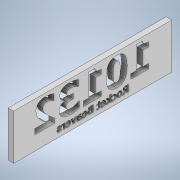
# Autodesk Inventor part: Vehicle Registration Plate
Saved by Autodesk Inventor 2020 (Build 240168000, 168)
## iProperties
Created: 2020-01-13
Part Number: Vehicle Registration Plate
Material: Generic
Document SubType Name: Modeling
Designer: maple
Density: 1 g/cm^3
Appearance: Default
Author: maple
Autodesk Inventor part; units mm, degrees
ref_plane "YZ Plane" through (0, 0, 0) normal (1, 0, 0) x (0, 1, 0)
ref_plane "XZ Plane" through (0, 0, 0) normal (0, 1, 0) x (-1, 0, 0)
ref_plane "XY Plane" through (0, 0, 0) normal (0, 0, 1) x (1, 0, 0)
sketch "Sketch1" plane through (0, 0, 0) normal (1, 0, 0) x (0, 1, 0)
  line L0 (0, 0) -> (-50.8, 0)
  line L1 (-50.8, 0) -> (-50.8, -177.8)
  line L2 (-50.8, -177.8) -> (0, -177.8)
  line L3 (0, -177.8) -> (0, 0)
  dimension "d0" = 50.8
  dimension "d1" = 177.8
  constraints: 8 end point, 2 parallel, 1 horizontal, 1 perpendicular
  measures "d0" distance of L2.end L1.end
  measures "d1" distance of L1.end L0.end
extrude "Extrusion1" add sketch "Sketch1" along normal blind 6.35
sketch "Sketch3" plane through (0, 0, 0) normal (-1, 0, 0) x (0, 0, 1)
  line L0 (-177.8, 0) -> (0, 0) projected
  line L1 (-88.9, 0) -> (-88.9, -50.8)
  line L2 (0, -50.8) -> (-177.8, -50.8) projected
  line L3 (-177.8, -50.8) -> (-177.8, 0) projected
  line L4 (-177.8, -25.4) -> (0, -25.4)
  line L5 (0, 0) -> (0, -50.8) projected
  line L6 (-172.4509, 0.5134) -> (-5.5704, 0.5134) construction
  line L7 (-5.5704, 0.5134) -> (-5.5704, -39.1921) construction
  line L8 (-5.5704, -39.1921) -> (-172.4509, -39.1921) construction
  line L9 (-172.4509, -39.1921) -> (-172.4509, 0.5134) construction
  line L10 (-156.8284, -35.0682) -> (-21.0393, -35.0682) construction
  line L11 (-21.0393, -35.0682) -> (-21.0393, -48.6327) construction
  line L12 (-21.0393, -48.6327) -> (-156.8284, -48.6327) construction
  line L13 (-156.8284, -48.6327) -> (-156.8284, -35.0682) construction
  line L14 (-131.6308, -34.5794) -> (-151.7614, -34.5794)
  line L15 (-151.7614, -34.5794) -> (-151.7614, -29.2688)
  line L16 (-151.7614, -29.2688) -> (-145.3394, -29.2688)
  line L17 (-145.3394, -29.2688) -> (-145.3394, -13.1396)
  line L18 (-145.3394, -13.1396) -> (-151.7614, -13.1396)
  line L19 (-151.7614, -13.1396) -> (-151.7614, -8.1749)
  spline S0 degree 2 poles (-151.7614, -8.1749) (-150.3535, -8.1749) (-147.5624, -7.8044) (-146.7226, -7.4092) knots 0 0 0 1 2 2 2
  spline S1 degree 2 poles (-146.7226, -7.4092) (-145.7593, -6.9152) (-144.6725, -5.2603) (-144.5737, -4.0253) knots 0 0 0 1 2 2 2
  line L20 (-144.5737, -4.0253) -> (-137.9046, -4.0253)
  line L21 (-137.9046, -4.0253) -> (-137.9046, -29.2688)
  line L22 (-137.9046, -29.2688) -> (-131.6308, -29.2688)
  line L23 (-131.6308, -29.2688) -> (-131.6308, -34.5794)
  spline S2 degree 2 poles (-103.9666, -19.3394) (-103.9666, -23.2914) (-105.2263, -29.2194) (-106.6342, -31.2201) knots 0 0 0 1 2 2 2
  spline S3 degree 2 poles (-106.6342, -31.2201) (-108.0174, -33.1962) (-112.4882, -35.2216) (-115.6992, -35.2216) knots 0 0 0 1 2 2 2
  spline S4 degree 2 poles (-115.6992, -35.2216) (-118.9349, -35.2216) (-123.3809, -33.1962) (-124.7889, -31.1707) knots 0 0 0 1 2 2 2
  spline S5 degree 2 poles (-124.7889, -31.1707) (-126.1968, -29.17) (-127.4565, -23.2914) (-127.4565, -19.3394) knots 0 0 0 1 2 2 2
  spline S6 degree 2 poles (-127.4565, -19.3394) (-127.4565, -15.2885) (-126.1968, -9.5581) (-124.7642, -7.4833) knots 0 0 0 1 2 2 2
  spline S7 degree 2 poles (-124.7642, -7.4833) (-123.3315, -5.4579) (-118.8114, -3.4819) (-115.6992, -3.4819) knots 0 0 0 1 2 2 2
  spline S8 degree 2 poles (-115.6992, -3.4819) (-112.4141, -3.4819) (-108.0174, -5.5567) (-106.6095, -7.6068) knots 0 0 0 1 2 2 2
  spline S9 degree 2 poles (-106.6095, -7.6068) (-105.2263, -9.6075) (-103.9666, -15.5108) (-103.9666, -19.3394) knots 0 0 0 1 2 2 2
  spline S10 degree 2 poles (-111.6484, -19.3394) (-111.6484, -13.683) (-113.5009, -9.1135) (-115.6992, -9.1135) knots 0 0 0 1 2 2 2
  spline S11 degree 2 poles (-115.6992, -9.1135) (-117.8975, -9.1135) (-119.7747, -13.683) (-119.7747, -19.3641) knots 0 0 0 1 2 2 2
  spline S12 degree 2 poles (-119.7747, -19.3641) (-119.7747, -24.9463) (-117.8975, -29.5899) (-115.6992, -29.5899) knots 0 0 0 1 2 2 2
  spline S13 degree 2 poles (-115.6992, -29.5899) (-113.5256, -29.5899) (-111.6484, -24.9463) (-111.6484, -19.3394) knots 0 0 0 1 2 2 2
  line L24 (-78.229, -34.5794) -> (-98.3597, -34.5794)
  line L25 (-98.3597, -34.5794) -> (-98.3597, -29.2688)
  line L26 (-98.3597, -29.2688) -> (-91.9376, -29.2688)
  line L27 (-91.9376, -29.2688) -> (-91.9376, -13.1396)
  line L28 (-91.9376, -13.1396) -> (-98.3597, -13.1396)
  line L29 (-98.3597, -13.1396) -> (-98.3597, -8.1749)
  spline S14 degree 2 poles (-98.3597, -8.1749) (-96.9518, -8.1749) (-94.1606, -7.8044) (-93.3208, -7.4092) knots 0 0 0 1 2 2 2
  spline S15 degree 2 poles (-93.3208, -7.4092) (-92.3575, -6.9152) (-91.2707, -5.2603) (-91.1719, -4.0253) knots 0 0 0 1 2 2 2
  line L30 (-91.1719, -4.0253) -> (-84.5029, -4.0253)
  line L31 (-84.5029, -4.0253) -> (-84.5029, -29.2688)
  line L32 (-84.5029, -29.2688) -> (-78.229, -29.2688)
  line L33 (-78.229, -29.2688) -> (-78.229, -34.5794)
  spline S16 degree 2 poles (-50.9354, -25.3415) (-50.9354, -27.5892) (-52.5903, -31.2695) (-54.1958, -32.5539) knots 0 0 0 1 2 2 2
  spline S17 degree 2 poles (-54.1958, -32.5539) (-55.8013, -33.8384) (-60.1732, -35.2216) (-63.3101, -35.2216) knots 0 0 0 1 2 2 2
  spline S18 degree 2 poles (-63.3101, -35.2216) (-66.867, -35.2216) (-71.9552, -34.036) (-73.5607, -33.295) knots 0 0 0 1 2 2 2
  line L34 (-73.5607, -33.295) -> (-73.5607, -26.6753)
  line L35 (-73.5607, -26.6753) -> (-72.8197, -26.6753)
  spline S19 degree 2 poles (-72.8197, -26.6753) (-71.1401, -27.7374) (-66.62, -29.3182) (-64.7428, -29.3182) knots 0 0 0 1 2 2 2
  spline S20 degree 2 poles (-64.7428, -29.3182) (-63.6312, -29.3182) (-61.0377, -28.923) (-60.1485, -28.2808) knots 0 0 0 1 2 2 2
  spline S21 degree 2 poles (-60.1485, -28.2808) (-59.4569, -27.7621) (-58.6171, -26.2554) (-58.6171, -24.8969) knots 0 0 0 1 2 2 2
  spline S22 degree 2 poles (-58.6171, -24.8969) (-58.6171, -23.5384) (-59.8027, -22.0811) (-60.7907, -21.7353) knots 0 0 0 1 2 2 2
  spline S23 degree 2 poles (-60.7907, -21.7353) (-61.7787, -21.3895) (-64.5205, -21.3154) (-65.5826, -21.3154) knots 0 0 0 1 2 2 2
  line L36 (-65.5826, -21.3154) -> (-66.8917, -21.3154)
  line L37 (-66.8917, -21.3154) -> (-66.8917, -15.9554)
  line L38 (-66.8917, -15.9554) -> (-65.6814, -15.9554)
  spline S24 degree 2 poles (-65.6814, -15.9554) (-64.2982, -15.9554) (-61.9516, -15.7084) (-61.1365, -15.3379) knots 0 0 0 1 2 2 2
  spline S25 degree 2 poles (-61.1365, -15.3379) (-60.3214, -14.9427) (-59.4075, -13.5595) (-59.4075, -12.3739) knots 0 0 0 1 2 2 2
  spline S26 degree 2 poles (-59.4075, -12.3739) (-59.4075, -11.4353) (-60.272, -10.2744) (-60.8895, -9.9533) knots 0 0 0 1 2 2 2
  spline S27 degree 2 poles (-60.8895, -9.9533) (-61.6305, -9.5828) (-63.6065, -9.3358) (-64.2982, -9.3358) knots 0 0 0 1 2 2 2
  spline S28 degree 2 poles (-64.2982, -9.3358) (-65.4097, -9.3358) (-67.7562, -9.8545) (-68.843, -10.2744) knots 0 0 0 1 2 2 2
  spline S29 degree 2 poles (-68.843, -10.2744) (-69.7075, -10.5955) (-71.5847, -11.6329) (-72.0293, -11.9046) knots 0 0 0 1 2 2 2
  line L39 (-72.0293, -11.9046) -> (-72.6715, -11.9046)
  line L40 (-72.6715, -11.9046) -> (-72.6715, -5.3838)
  spline S30 degree 2 poles (-72.6715, -5.3838) (-71.0907, -4.7169) (-65.7555, -3.4572) (-62.9643, -3.4572) knots 0 0 0 1 2 2 2
  spline S31 degree 2 poles (-62.9643, -3.4572) (-60.2473, -3.4572) (-56.2459, -4.3958) (-54.838, -5.3097) knots 0 0 0 1 2 2 2
  spline S32 degree 2 poles (-54.838, -5.3097) (-53.2819, -6.273) (-51.7258, -9.237) (-51.7258, -11.0895) knots 0 0 0 1 2 2 2
  spline S33 degree 2 poles (-51.7258, -11.0895) (-51.7258, -13.7077) (-54.7392, -17.6104) (-57.2092, -18.1785) knots 0 0 0 1 2 2 2
  line L41 (-57.2092, -18.1785) -> (-57.2092, -18.4749)
  spline S34 degree 2 poles (-57.2092, -18.4749) (-56.1224, -18.6231) (-54.0476, -19.4135) (-53.0596, -20.3027) knots 0 0 0 1 2 2 2
  spline S35 degree 2 poles (-53.0596, -20.3027) (-52.1457, -21.0931) (-50.9354, -23.6125) (-50.9354, -25.3415) knots 0 0 0 1 2 2 2
  line L42 (-23.4688, -34.5794) -> (-45.8718, -34.5794)
  line L43 (-45.8718, -34.5794) -> (-45.8718, -29.6146)
  spline S36 degree 2 poles (-45.8718, -29.6146) (-43.0313, -27.3422) (-38.4865, -23.3408) (-36.7822, -21.5377) knots 0 0 0 1 2 2 2
  spline S37 degree 2 poles (-36.7822, -21.5377) (-34.5345, -19.1912) (-32.5337, -15.6096) (-32.5337, -13.7324) knots 0 0 0 1 2 2 2
  spline S38 degree 2 poles (-32.5337, -13.7324) (-32.5337, -11.6082) (-35.0779, -9.3358) (-37.3503, -9.3358) knots 0 0 0 1 2 2 2
  spline S39 degree 2 poles (-37.3503, -9.3358) (-38.5112, -9.3358) (-40.586, -9.9039) (-41.6481, -10.3485) knots 0 0 0 1 2 2 2
  spline S40 degree 2 poles (-41.6481, -10.3485) (-42.6855, -10.8178) (-44.1675, -11.8058) (-44.538, -12.0528) knots 0 0 0 1 2 2 2
  line L44 (-44.538, -12.0528) -> (-45.1308, -12.0528)
  line L45 (-45.1308, -12.0528) -> (-45.1308, -5.4085)
  spline S41 degree 2 poles (-45.1308, -5.4085) (-43.8464, -4.791) (-38.363, -3.5066) (-35.8189, -3.5066) knots 0 0 0 1 2 2 2
  spline S42 degree 2 poles (-35.8189, -3.5066) (-30.3848, -3.5066) (-24.8026, -8.3478) (-24.8026, -12.7197) knots 0 0 0 1 2 2 2
  spline S43 degree 2 poles (-24.8026, -12.7197) (-24.8026, -15.412) (-27.3467, -20.5991) (-30.286, -23.5631) knots 0 0 0 1 2 2 2
  spline S44 degree 2 poles (-30.286, -23.5631) (-32.1385, -25.3909) (-35.6213, -28.2314) (-36.387, -28.8242) knots 0 0 0 1 2 2 2
  line L46 (-36.387, -28.8242) -> (-23.4688, -28.8242)
  line L47 (-23.4688, -28.8242) -> (-23.4688, -34.5794)
  line L48 (-121.8406, -45.7407) -> (-124.1686, -45.7407)
  line L49 (-124.1686, -45.7407) -> (-126.2866, -42.9434)
  line L50 (-126.2866, -42.9434) -> (-126.9783, -42.9434)
  line L51 (-126.9783, -42.9434) -> (-126.9783, -45.7407)
  line L52 (-126.9783, -45.7407) -> (-128.8802, -45.7407)
  line L53 (-128.8802, -45.7407) -> (-128.8802, -38.1207)
  line L54 (-128.8802, -38.1207) -> (-125.8173, -38.1207)
  spline S45 degree 2 poles (-125.8173, -38.1207) (-125.1813, -38.1207) (-124.2427, -38.2813) (-123.8413, -38.5283) knots 0 0 0 1 2 2 2
  spline S46 degree 2 poles (-123.8413, -38.5283) (-123.4338, -38.7876) (-122.9521, -39.5965) (-122.9521, -40.214) knots 0 0 0 1 2 2 2
  spline S47 degree 2 poles (-122.9521, -40.214) (-122.9521, -41.0847) (-123.7425, -42.1777) (-124.4033, -42.4988) knots 0 0 0 1 2 2 2
  line L55 (-124.4033, -42.4988) -> (-121.8406, -45.7407)
  spline S48 degree 2 poles (-124.9158, -40.4549) (-124.9158, -40.1646) (-125.1381, -39.7509) (-125.3913, -39.6398) knots 0 0 0 1 2 2 2
  spline S49 degree 2 poles (-125.3913, -39.6398) (-125.5703, -39.5657) (-126.0088, -39.5224) (-126.336, -39.5224) knots 0 0 0 1 2 2 2
  line L56 (-126.336, -39.5224) -> (-126.9783, -39.5224)
  line L57 (-126.9783, -39.5224) -> (-126.9783, -41.5726)
  line L58 (-126.9783, -41.5726) -> (-126.4287, -41.5726)
  spline S50 degree 2 poles (-126.4287, -41.5726) (-126.0335, -41.5726) (-125.4715, -41.4737) (-125.2801, -41.3194) knots 0 0 0 1 2 2 2
  spline S51 degree 2 poles (-125.2801, -41.3194) (-125.0949, -41.1712) (-124.9158, -40.776) (-124.9158, -40.4549) knots 0 0 0 1 2 2 2
  spline S52 degree 2 poles (-115.8632, -42.8693) (-115.8632, -44.2896) (-117.4131, -45.9198) (-118.8272, -45.9198) knots 0 0 0 1 2 2 2
  spline S53 degree 2 poles (-118.8272, -45.9198) (-120.2351, -45.9198) (-121.7974, -44.2896) (-121.7974, -42.8693) knots 0 0 0 1 2 2 2
  spline S54 degree 2 poles (-121.7974, -42.8693) (-121.7974, -41.4367) (-120.2351, -39.8127) (-118.8272, -39.8127) knots 0 0 0 1 2 2 2
  spline S55 degree 2 poles (-118.8272, -39.8127) (-117.4193, -39.8127) (-115.8632, -41.4429) (-115.8632, -42.8693) knots 0 0 0 1 2 2 2
  spline S56 degree 2 poles (-117.6972, -42.8817) (-117.6972, -42.3691) (-117.8639, -41.6837) (-118.0121, -41.4799) knots 0 0 0 1 2 2 2
  spline S57 degree 2 poles (-118.0121, -41.4799) (-118.1726, -41.2638) (-118.574, -41.0971) (-118.8272, -41.0971) knots 0 0 0 1 2 2 2
  spline S58 degree 2 poles (-118.8272, -41.0971) (-119.0742, -41.0971) (-119.4632, -41.2453) (-119.6238, -41.4552) knots 0 0 0 1 2 2 2
  spline S59 degree 2 poles (-119.6238, -41.4552) (-119.7782, -41.6528) (-119.9634, -42.3506) (-119.9634, -42.8817) knots 0 0 0 1 2 2 2
  spline S60 degree 2 poles (-119.9634, -42.8817) (-119.9634, -43.4065) (-119.7905, -44.0549) (-119.6485, -44.2525) knots 0 0 0 1 2 2 2
  spline S61 degree 2 poles (-119.6485, -44.2525) (-119.5065, -44.4501) (-119.0742, -44.6354) (-118.8148, -44.6354) knots 0 0 0 1 2 2 2
  spline S62 degree 2 poles (-118.8148, -44.6354) (-118.5987, -44.6354) (-118.1541, -44.4501) (-118.0183, -44.2649) knots 0 0 0 1 2 2 2
  spline S63 degree 2 poles (-118.0183, -44.2649) (-117.8639, -44.0487) (-117.6972, -43.4251) (-117.6972, -42.8817) knots 0 0 0 1 2 2 2
  spline S64 degree 2 poles (-112.0964, -45.8951) (-112.8065, -45.8951) (-113.986, -45.5369) (-114.4244, -45.1664) knots 0 0 0 1 2 2 2
  spline S65 degree 2 poles (-114.4244, -45.1664) (-114.8505, -44.7897) (-115.3321, -43.6597) (-115.3321, -42.894) knots 0 0 0 1 2 2 2
  spline S66 degree 2 poles (-115.3321, -42.894) (-115.3321, -42.0666) (-114.8134, -40.9118) (-114.3626, -40.5413) knots 0 0 0 1 2 2 2
  spline S67 degree 2 poles (-114.3626, -40.5413) (-113.9366, -40.1832) (-112.7757, -39.8374) (-112.1458, -39.8374) knots 0 0 0 1 2 2 2
  spline S68 degree 2 poles (-112.1458, -39.8374) (-111.6703, -39.8374) (-110.7194, -40.0597) (-110.2377, -40.3005) knots 0 0 0 1 2 2 2
  line L59 (-110.2377, -40.3005) -> (-110.2377, -41.8319)
  line L60 (-110.2377, -41.8319) -> (-110.4662, -41.8319)
  spline S69 degree 2 poles (-110.4662, -41.8319) (-110.5773, -41.7269) (-110.8861, -41.4799) (-111.0713, -41.3811) knots 0 0 0 1 2 2 2
  spline S70 degree 2 poles (-111.0713, -41.3811) (-111.2689, -41.27) (-111.7568, -41.1218) (-112.0594, -41.1218) knots 0 0 0 1 2 2 2
  spline S71 degree 2 poles (-112.0594, -41.1218) (-112.7448, -41.1218) (-113.4981, -42.0789) (-113.4981, -42.894) knots 0 0 0 1 2 2 2
  spline S72 degree 2 poles (-113.4981, -42.894) (-113.4981, -43.7585) (-112.6954, -44.6107) (-112.0285, -44.6107) knots 0 0 0 1 2 2 2
  spline S73 degree 2 poles (-112.0285, -44.6107) (-111.6889, -44.6107) (-111.1825, -44.4563) (-110.9972, -44.3451) knots 0 0 0 1 2 2 2
  spline S74 degree 2 poles (-110.9972, -44.3451) (-110.8182, -44.2402) (-110.5588, -44.0055) (-110.4662, -43.9129) knots 0 0 0 1 2 2 2
  line L61 (-110.4662, -43.9129) -> (-110.2377, -43.9129)
  line L62 (-110.2377, -43.9129) -> (-110.2377, -45.4505)
  spline S75 degree 2 poles (-110.2377, -45.4505) (-110.3921, -45.5184) (-110.7935, -45.6913) (-111.0034, -45.7469) knots 0 0 0 1 2 2 2
  spline S76 degree 2 poles (-111.0034, -45.7469) (-111.2628, -45.821) (-111.7197, -45.8951) (-112.0964, -45.8951) knots 0 0 0 1 2 2 2
  line L63 (-103.6304, -45.7407) -> (-105.7608, -45.7407)
  line L64 (-105.7608, -45.7407) -> (-107.3169, -43.246)
  line L65 (-107.3169, -43.246) -> (-107.5948, -43.6165)
  line L66 (-107.5948, -43.6165) -> (-107.5948, -45.7407)
  line L67 (-107.5948, -45.7407) -> (-109.3856, -45.7407)
  line L68 (-109.3856, -45.7407) -> (-109.3856, -37.7811)
  line L69 (-109.3856, -37.7811) -> (-107.5948, -37.7811)
  line L70 (-107.5948, -37.7811) -> (-107.5948, -42.2395)
  line L71 (-107.5948, -42.2395) -> (-105.8967, -39.9917)
  line L72 (-105.8967, -39.9917) -> (-103.7786, -39.9917)
  line L73 (-103.7786, -39.9917) -> (-105.7917, -42.4679)
  line L74 (-105.7917, -42.4679) -> (-103.6304, -45.7407)
  spline S77 degree 2 poles (-100.123, -45.8951) (-101.7532, -45.8951) (-103.4884, -44.339) (-103.4884, -42.9002) knots 0 0 0 1 2 2 2
  spline S78 degree 2 poles (-103.4884, -42.9002) (-103.4884, -41.4923) (-101.8705, -39.8127) (-100.4132, -39.8127) knots 0 0 0 1 2 2 2
  spline S79 degree 2 poles (-100.4132, -39.8127) (-99.0979, -39.8127) (-97.7641, -41.2391) (-97.7641, -42.5606) knots 0 0 0 1 2 2 2
  line L75 (-97.7641, -42.5606) -> (-97.7641, -43.2089)
  line L76 (-97.7641, -43.2089) -> (-101.6976, -43.2089)
  spline S80 degree 2 poles (-101.6976, -43.2089) (-101.6729, -43.6103) (-101.3827, -44.1414) (-101.1481, -44.3019) knots 0 0 0 1 2 2 2
  spline S81 degree 2 poles (-101.1481, -44.3019) (-100.9196, -44.4625) (-100.3021, -44.5983) (-99.9377, -44.5983) knots 0 0 0 1 2 2 2
  spline S82 degree 2 poles (-99.9377, -44.5983) (-99.629, -44.5983) (-99.0238, -44.4625) (-98.7707, -44.3451) knots 0 0 0 1 2 2 2
  spline S83 degree 2 poles (-98.7707, -44.3451) (-98.5484, -44.2525) (-98.1779, -44.024) (-98.0605, -43.9376) knots 0 0 0 1 2 2 2
  line L77 (-98.0605, -43.9376) -> (-97.8691, -43.9376)
  line L78 (-97.8691, -43.9376) -> (-97.8691, -45.4196)
  spline S84 degree 2 poles (-97.8691, -45.4196) (-98.0914, -45.5061) (-98.4496, -45.6543) (-98.7707, -45.7284) knots 0 0 0 1 2 2 2
  spline S85 degree 2 poles (-98.7707, -45.7284) (-99.0609, -45.8086) (-99.6784, -45.8951) (-100.123, -45.8951) knots 0 0 0 1 2 2 2
  spline S86 degree 2 poles (-99.5302, -42.1283) (-99.5425, -41.5602) (-100.0427, -40.9612) (-100.5553, -40.9612) knots 0 0 0 1 2 2 2
  spline S87 degree 2 poles (-100.5553, -40.9612) (-101.0801, -40.9612) (-101.6729, -41.5911) (-101.7038, -42.1283) knots 0 0 0 1 2 2 2
  line L79 (-101.7038, -42.1283) -> (-99.5302, -42.1283)
  spline S88 degree 2 poles (-94.6457, -45.8519) (-95.7387, -45.8519) (-96.7391, -44.9503) (-96.7391, -43.9252) knots 0 0 0 1 2 2 2
  line L80 (-96.7391, -43.9252) -> (-96.7391, -41.2391)
  line L81 (-96.7391, -41.2391) -> (-97.4245, -41.2391)
  line L82 (-97.4245, -41.2391) -> (-97.4245, -39.9917)
  line L83 (-97.4245, -39.9917) -> (-96.7391, -39.9917)
  line L84 (-96.7391, -39.9917) -> (-96.7391, -38.3492)
  line L85 (-96.7391, -38.3492) -> (-94.9483, -38.3492)
  line L86 (-94.9483, -38.3492) -> (-94.9483, -39.9917)
  line L87 (-94.9483, -39.9917) -> (-93.2193, -39.9917)
  line L88 (-93.2193, -39.9917) -> (-93.2193, -41.2391)
  line L89 (-93.2193, -41.2391) -> (-94.9483, -41.2391)
  line L90 (-94.9483, -41.2391) -> (-94.9483, -43.283)
  spline S89 degree 2 poles (-94.9483, -43.283) (-94.9483, -43.5856) (-94.936, -44.0364) (-94.8619, -44.2155) knots 0 0 0 1 2 2 2
  spline S90 degree 2 poles (-94.8619, -44.2155) (-94.7878, -44.3945) (-94.4234, -44.6045) (-94.0776, -44.6045) knots 0 0 0 1 2 2 2
  spline S91 degree 2 poles (-94.0776, -44.6045) (-93.9294, -44.6045) (-93.4663, -44.481) (-93.3737, -44.4316) knots 0 0 0 1 2 2 2
  line L91 (-93.3737, -44.4316) -> (-93.2193, -44.4316)
  line L92 (-93.2193, -44.4316) -> (-93.2193, -45.6913)
  spline S92 degree 2 poles (-93.2193, -45.6913) (-93.5095, -45.7654) (-94.1641, -45.8519) (-94.6457, -45.8519) knots 0 0 0 1 2 2 2
  spline S93 degree 2 poles (-83.2281, -43.4065) (-83.2281, -43.9746) (-83.6603, -44.833) (-84.0185, -45.117) knots 0 0 0 1 2 2 2
  spline S94 degree 2 poles (-84.0185, -45.117) (-84.4507, -45.4567) (-85.4758, -45.7407) (-86.2724, -45.7407) knots 0 0 0 1 2 2 2
  line L93 (-86.2724, -45.7407) -> (-89.3167, -45.7407)
  line L94 (-89.3167, -45.7407) -> (-89.3167, -38.1207)
  line L95 (-89.3167, -38.1207) -> (-86.6305, -38.1207)
  spline S95 degree 2 poles (-86.6305, -38.1207) (-85.7907, -38.1207) (-84.9262, -38.2504) (-84.5495, -38.4542) knots 0 0 0 1 2 2 2
  spline S96 degree 2 poles (-84.5495, -38.4542) (-84.1358, -38.6703) (-83.7344, -39.4113) (-83.7344, -39.8929) knots 0 0 0 1 2 2 2
  spline S97 degree 2 poles (-83.7344, -39.8929) (-83.7344, -40.4487) (-84.2902, -41.3194) (-84.7842, -41.5231) knots 0 0 0 1 2 2 2
  line L96 (-84.7842, -41.5231) -> (-84.7842, -41.5602)
  spline S98 degree 2 poles (-84.7842, -41.5602) (-84.0741, -41.7084) (-83.2281, -42.6285) (-83.2281, -43.4065) knots 0 0 0 1 2 2 2
  spline S99 degree 2 poles (-85.2041, -43.3757) (-85.2041, -43.0175) (-85.4882, -42.6161) (-85.7722, -42.5112) knots 0 0 0 1 2 2 2
  spline S100 degree 2 poles (-85.7722, -42.5112) (-85.9451, -42.4432) (-86.5564, -42.4309) (-87.0628, -42.4309) knots 0 0 0 1 2 2 2
  line L97 (-87.0628, -42.4309) -> (-87.4148, -42.4309)
  line L98 (-87.4148, -42.4309) -> (-87.4148, -44.3513)
  line L99 (-87.4148, -44.3513) -> (-87.3098, -44.3513)
  spline S101 degree 2 poles (-87.3098, -44.3513) (-86.5688, -44.3513) (-86.0007, -44.3328) (-85.7043, -44.2031) knots 0 0 0 1 2 2 2
  spline S102 degree 2 poles (-85.7043, -44.2031) (-85.4449, -44.0858) (-85.2041, -43.6535) (-85.2041, -43.3757) knots 0 0 0 1 2 2 2
  spline S103 degree 2 poles (-85.6796, -40.2696) (-85.6796, -40.0844) (-85.871, -39.6953) (-86.0686, -39.6089) knots 0 0 0 1 2 2 2
  spline S104 degree 2 poles (-86.0686, -39.6089) (-86.2539, -39.5224) (-86.7726, -39.5101) (-87.2851, -39.5101) knots 0 0 0 1 2 2 2
  line L100 (-87.2851, -39.5101) -> (-87.4148, -39.5101)
  line L101 (-87.4148, -39.5101) -> (-87.4148, -41.1279)
  line L102 (-87.4148, -41.1279) -> (-87.1739, -41.1279)
  spline S105 degree 2 poles (-87.1739, -41.1279) (-86.6861, -41.1279) (-86.2909, -41.1094) (-86.081, -41.0106) knots 0 0 0 1 2 2 2
  spline S106 degree 2 poles (-86.081, -41.0106) (-85.8525, -40.8995) (-85.6796, -40.5228) (-85.6796, -40.2696) knots 0 0 0 1 2 2 2
  spline S107 degree 2 poles (-79.2884, -45.8951) (-80.9186, -45.8951) (-82.6538, -44.339) (-82.6538, -42.9002) knots 0 0 0 1 2 2 2
  spline S108 degree 2 poles (-82.6538, -42.9002) (-82.6538, -41.4923) (-81.0359, -39.8127) (-79.5786, -39.8127) knots 0 0 0 1 2 2 2
  spline S109 degree 2 poles (-79.5786, -39.8127) (-78.2634, -39.8127) (-76.9295, -41.2391) (-76.9295, -42.5606) knots 0 0 0 1 2 2 2
  line L103 (-76.9295, -42.5606) -> (-76.9295, -43.2089)
  line L104 (-76.9295, -43.2089) -> (-80.863, -43.2089)
  spline S110 degree 2 poles (-80.863, -43.2089) (-80.8383, -43.6103) (-80.5481, -44.1414) (-80.3135, -44.3019) knots 0 0 0 1 2 2 2
  spline S111 degree 2 poles (-80.3135, -44.3019) (-80.085, -44.4625) (-79.4675, -44.5983) (-79.1032, -44.5983) knots 0 0 0 1 2 2 2
  spline S112 degree 2 poles (-79.1032, -44.5983) (-78.7944, -44.5983) (-78.1893, -44.4625) (-77.9361, -44.3451) knots 0 0 0 1 2 2 2
  spline S113 degree 2 poles (-77.9361, -44.3451) (-77.7138, -44.2525) (-77.3433, -44.024) (-77.2259, -43.9376) knots 0 0 0 1 2 2 2
  line L105 (-77.2259, -43.9376) -> (-77.0345, -43.9376)
  line L106 (-77.0345, -43.9376) -> (-77.0345, -45.4196)
  spline S114 degree 2 poles (-77.0345, -45.4196) (-77.2568, -45.5061) (-77.615, -45.6543) (-77.9361, -45.7284) knots 0 0 0 1 2 2 2
  spline S115 degree 2 poles (-77.9361, -45.7284) (-78.2263, -45.8086) (-78.8438, -45.8951) (-79.2884, -45.8951) knots 0 0 0 1 2 2 2
  spline S116 degree 2 poles (-78.6956, -42.1283) (-78.708, -41.5602) (-79.2081, -40.9612) (-79.7207, -40.9612) knots 0 0 0 1 2 2 2
  spline S117 degree 2 poles (-79.7207, -40.9612) (-80.2455, -40.9612) (-80.8383, -41.5911) (-80.8692, -42.1283) knots 0 0 0 1 2 2 2
  line L107 (-80.8692, -42.1283) -> (-78.6956, -42.1283)
  spline S118 degree 2 poles (-72.8417, -45.1294) (-73.0269, -45.2837) (-73.3171, -45.5308) (-73.5642, -45.6543) knots 0 0 0 1 2 2 2
  spline S119 degree 2 poles (-73.5642, -45.6543) (-73.805, -45.7716) (-74.2619, -45.8951) (-74.6695, -45.8951) knots 0 0 0 1 2 2 2
  spline S120 degree 2 poles (-74.6695, -45.8951) (-75.4352, -45.8951) (-76.4417, -44.87) (-76.4417, -44.092) knots 0 0 0 1 2 2 2
  spline S121 degree 2 poles (-76.4417, -44.092) (-76.4417, -43.4559) (-75.9292, -42.6655) (-75.4475, -42.4371) knots 0 0 0 1 2 2 2
  spline S122 degree 2 poles (-75.4475, -42.4371) (-74.9597, -42.2024) (-73.6074, -42.0172) (-72.8293, -41.9678) knots 0 0 0 1 2 2 2
  line L108 (-72.8293, -41.9678) -> (-72.8293, -41.9369)
  spline S123 degree 2 poles (-72.8293, -41.9369) (-72.8293, -41.4614) (-73.5333, -41.0971) (-74.2372, -41.0971) knots 0 0 0 1 2 2 2
  spline S124 degree 2 poles (-74.2372, -41.0971) (-74.5522, -41.0971) (-75.4043, -41.3255) (-75.8057, -41.5046) knots 0 0 0 1 2 2 2
  line L109 (-75.8057, -41.5046) -> (-75.9601, -41.5046)
  line L110 (-75.9601, -41.5046) -> (-75.9601, -40.1152)
  spline S125 degree 2 poles (-75.9601, -40.1152) (-75.6945, -40.0411) (-74.5089, -39.8312) (-73.9038, -39.8312) knots 0 0 0 1 2 2 2
  spline S126 degree 2 poles (-73.9038, -39.8312) (-72.4218, -39.8312) (-71.0633, -40.8192) (-71.0633, -41.8319) knots 0 0 0 1 2 2 2
  line L111 (-71.0633, -41.8319) -> (-71.0633, -45.7407)
  line L112 (-71.0633, -45.7407) -> (-72.8417, -45.7407)
  line L113 (-72.8417, -45.7407) -> (-72.8417, -45.1294)
  line L114 (-72.8417, -44.2402) -> (-72.8417, -43.0484)
  spline S127 degree 2 poles (-72.8417, -43.0484) (-73.2986, -43.0916) (-73.8606, -43.1595) (-74.1323, -43.2583) knots 0 0 0 1 2 2 2
  spline S128 degree 2 poles (-74.1323, -43.2583) (-74.3731, -43.3386) (-74.6324, -43.6721) (-74.6324, -43.9438) knots 0 0 0 1 2 2 2
  spline S129 degree 2 poles (-74.6324, -43.9438) (-74.6324, -44.3451) (-74.194, -44.6477) (-73.7679, -44.6477) knots 0 0 0 1 2 2 2
  spline S130 degree 2 poles (-73.7679, -44.6477) (-73.5333, -44.6477) (-73.0393, -44.4316) (-72.8417, -44.2402) knots 0 0 0 1 2 2 2
  line L115 (-64.3572, -39.9917) -> (-66.4196, -45.7407)
  line L116 (-66.4196, -45.7407) -> (-68.3771, -45.7407)
  line L117 (-68.3771, -45.7407) -> (-70.4211, -39.9917)
  line L118 (-70.4211, -39.9917) -> (-68.5377, -39.9917)
  line L119 (-68.5377, -39.9917) -> (-67.3644, -43.7894)
  line L120 (-67.3644, -43.7894) -> (-66.2035, -39.9917)
  line L121 (-66.2035, -39.9917) -> (-64.3572, -39.9917)
  spline S131 degree 2 poles (-60.7262, -45.8951) (-62.3565, -45.8951) (-64.0916, -44.339) (-64.0916, -42.9002) knots 0 0 0 1 2 2 2
  spline S132 degree 2 poles (-64.0916, -42.9002) (-64.0916, -41.4923) (-62.4738, -39.8127) (-61.0165, -39.8127) knots 0 0 0 1 2 2 2
  spline S133 degree 2 poles (-61.0165, -39.8127) (-59.7012, -39.8127) (-58.3674, -41.2391) (-58.3674, -42.5606) knots 0 0 0 1 2 2 2
  line L122 (-58.3674, -42.5606) -> (-58.3674, -43.2089)
  line L123 (-58.3674, -43.2089) -> (-62.3009, -43.2089)
  spline S134 degree 2 poles (-62.3009, -43.2089) (-62.2762, -43.6103) (-61.9859, -44.1414) (-61.7513, -44.3019) knots 0 0 0 1 2 2 2
  spline S135 degree 2 poles (-61.7513, -44.3019) (-61.5228, -44.4625) (-60.9053, -44.5983) (-60.541, -44.5983) knots 0 0 0 1 2 2 2
  spline S136 degree 2 poles (-60.541, -44.5983) (-60.2322, -44.5983) (-59.6271, -44.4625) (-59.3739, -44.3451) knots 0 0 0 1 2 2 2
  spline S137 degree 2 poles (-59.3739, -44.3451) (-59.1516, -44.2525) (-58.7811, -44.024) (-58.6638, -43.9376) knots 0 0 0 1 2 2 2
  line L124 (-58.6638, -43.9376) -> (-58.4724, -43.9376)
  line L125 (-58.4724, -43.9376) -> (-58.4724, -45.4196)
  spline S138 degree 2 poles (-58.4724, -45.4196) (-58.6947, -45.5061) (-59.0528, -45.6543) (-59.3739, -45.7284) knots 0 0 0 1 2 2 2
  spline S139 degree 2 poles (-59.3739, -45.7284) (-59.6641, -45.8086) (-60.2816, -45.8951) (-60.7262, -45.8951) knots 0 0 0 1 2 2 2
  spline S140 degree 2 poles (-60.1334, -42.1283) (-60.1458, -41.5602) (-60.646, -40.9612) (-61.1585, -40.9612) knots 0 0 0 1 2 2 2
  spline S141 degree 2 poles (-61.1585, -40.9612) (-61.6834, -40.9612) (-62.2762, -41.5911) (-62.3071, -42.1283) knots 0 0 0 1 2 2 2
  line L126 (-62.3071, -42.1283) -> (-60.1334, -42.1283)
  line L127 (-53.5879, -41.6899) -> (-53.7361, -41.6899)
  spline S142 degree 2 poles (-53.7361, -41.6899) (-53.8411, -41.6528) (-54.2301, -41.6158) (-54.4647, -41.6158) knots 0 0 0 1 2 2 2
  spline S143 degree 2 poles (-54.4647, -41.6158) (-54.7426, -41.6158) (-55.3663, -41.7825) (-55.6565, -41.8937) knots 0 0 0 1 2 2 2
  line L128 (-55.6565, -41.8937) -> (-55.6565, -45.7407)
  line L129 (-55.6565, -45.7407) -> (-57.4473, -45.7407)
  line L130 (-57.4473, -45.7407) -> (-57.4473, -39.9917)
  line L131 (-57.4473, -39.9917) -> (-55.6565, -39.9917)
  line L132 (-55.6565, -39.9917) -> (-55.6565, -40.8192)
  spline S144 degree 2 poles (-55.6565, -40.8192) (-55.533, -40.708) (-55.1008, -40.3622) (-54.9217, -40.2573) knots 0 0 0 1 2 2 2
  spline S145 degree 2 poles (-54.9217, -40.2573) (-54.7241, -40.1399) (-54.2054, -39.9732) (-53.9769, -39.9732) knots 0 0 0 1 2 2 2
  spline S146 degree 2 poles (-53.9769, -39.9732) (-53.8905, -39.9732) (-53.6743, -39.9856) (-53.5879, -39.9917) knots 0 0 0 1 2 2 2
  line L133 (-53.5879, -39.9917) -> (-53.5879, -41.6899)
  spline S147 degree 2 poles (-51.1549, -45.8951) (-51.7848, -45.8951) (-52.9148, -45.6172) (-53.2853, -45.432) knots 0 0 0 1 2 2 2
  line L134 (-53.2853, -45.432) -> (-53.2853, -43.9191)
  line L135 (-53.2853, -43.9191) -> (-53.1371, -43.9191)
  spline S148 degree 2 poles (-53.1371, -43.9191) (-53.0074, -44.0179) (-52.6802, -44.2525) (-52.3899, -44.3822) knots 0 0 0 1 2 2 2
  spline S149 degree 2 poles (-52.3899, -44.3822) (-52.1368, -44.4995) (-51.5131, -44.6662) (-51.1426, -44.6662) knots 0 0 0 1 2 2 2
  spline S150 degree 2 poles (-51.1426, -44.6662) (-50.7659, -44.6662) (-50.1854, -44.4316) (-50.1854, -44.1784) knots 0 0 0 1 2 2 2
  spline S151 degree 2 poles (-50.1854, -44.1784) (-50.1854, -43.9808) (-50.451, -43.7709) (-50.8338, -43.6844) knots 0 0 0 1 2 2 2
  spline S152 degree 2 poles (-50.8338, -43.6844) (-51.0376, -43.6288) (-51.6613, -43.5115) (-51.9021, -43.4374) knots 0 0 0 1 2 2 2
  spline S153 degree 2 poles (-51.9021, -43.4374) (-52.5814, -43.2275) (-53.2606, -42.4062) (-53.2606, -41.7331) knots 0 0 0 1 2 2 2
  spline S154 degree 2 poles (-53.2606, -41.7331) (-53.2606, -41.3502) (-52.9086, -40.671) (-52.5628, -40.4055) knots 0 0 0 1 2 2 2
  spline S155 degree 2 poles (-52.5628, -40.4055) (-52.2232, -40.1461) (-51.2167, -39.8374) (-50.5806, -39.8374) knots 0 0 0 1 2 2 2
  spline S156 degree 2 poles (-50.5806, -39.8374) (-49.9755, -39.8374) (-48.9628, -40.0782) (-48.617, -40.2449) knots 0 0 0 1 2 2 2
  line L136 (-48.617, -40.2449) -> (-48.617, -41.7022)
  line L137 (-48.617, -41.7022) -> (-48.759, -41.7022)
  spline S157 degree 2 poles (-48.759, -41.7022) (-48.8516, -41.6281) (-49.253, -41.3873) (-49.4383, -41.3008) knots 0 0 0 1 2 2 2
  spline S158 degree 2 poles (-49.4383, -41.3008) (-49.6667, -41.202) (-50.2225, -41.0662) (-50.5127, -41.0662) knots 0 0 0 1 2 2 2
  spline S159 degree 2 poles (-50.5127, -41.0662) (-50.9018, -41.0662) (-51.439, -41.3317) (-51.439, -41.5478) knots 0 0 0 1 2 2 2
  spline S160 degree 2 poles (-51.439, -41.5478) (-51.439, -41.7455) (-51.1735, -41.9678) (-50.7288, -42.0789) knots 0 0 0 1 2 2 2
  spline S161 degree 2 poles (-50.7288, -42.0789) (-50.5004, -42.1345) (-49.9014, -42.2395) (-49.6235, -42.3321) knots 0 0 0 1 2 2 2
  spline S162 degree 2 poles (-49.6235, -42.3321) (-49.006, -42.5297) (-48.3638, -43.3016) (-48.3638, -43.9438) knots 0 0 0 1 2 2 2
  spline S163 degree 2 poles (-48.3638, -43.9438) (-48.3638, -44.3451) (-48.7405, -45.08) (-49.0925, -45.327) knots 0 0 0 1 2 2 2
  spline S164 degree 2 poles (-49.0925, -45.327) (-49.4568, -45.5987) (-50.4571, -45.8951) (-51.1549, -45.8951) knots 0 0 0 1 2 2 2
  constraints: 4 end point, 4 midpoint, 4 other
emboss "Emboss1" sketch "Sketch3" operation cut depth 6.35 direction (1, 0, 0) contours L30 L31 L4 L1 | L1 L4 L27 L28 L29 S14 S15 L30 | L17 L18 L19 S0 S1 L20 L21 L4 | L4 L21 L22 L23 L14 L15 L16 L17 | L4 L31 L32 L33 L24 L1 | L1 L24 L25 L26 L27 L4 | S44 L46 L47 L42 L43 S36 L4 | L4 S36 S37 S38 S39 S40 L44 L45 S41 S42 S43 S44 | L93 L94 L95 L1 | L1 L95 S95 S96 S97 L96 S98 S93 S94 L93 | S5 S6 S7 S8 S9 S2 L4 S13 S10 S11 S12 | L4 S12 S13 S2 S3 S4 S5 | S21 S22 S23 L36 L37 L38 S24 S25 S26 S27 S28 S29 L39 L40 S30 S31 S32 S33 L41 S34 S35 S16 L4 | L4 S16 S17 S18 L34 L35 S19 S20 S21 | L48 L49 L50 L51 L52 L53 L54 S45 S46 S47 L55 | S52 S53 S54 S55 | S64 S65 S66 S67 S68 L59 L60 S69 S70 S71 S72 S73 S74 L61 L62 S75 S76 | L63 L64 L65 L66 L67 L68 L69 L70 L71 L72 L73 L74 | S77 S78 S79 L75 L76 S80 S81 S82 S83 L77 L78 S84 S85 | S88 L80 L81 L82 L83 L84 L85 L86 L87 L88 L89 L90 S89 S90 S91 L91 L92 S92 | S107 S108 S109 L103 L104 S110 S111 S112 S113 L105 L106 S114 S115 | S118 S119 S120 S121 S122 L108 S123 S124 L109 L110 S125 S126 L111 L112 L113 | L115 L116 L117 L118 L119 L120 L121 | S131 S132 S133 L122 L123 S134 S135 S136 S137 L124 L125 S138 S139 | L127 S142 S143 L128 L129 L130 L131 L132 S144 S145 S146 L133 | S147 L134 L135 S148 S149 S150 S151 S152 S153 S154 S155 S156 L136 L137 S157 S158 S159 S160 S161 S162 S163 S164
body "Solid1"
